Autodesk Fusion 360 part; units mm, degrees
(part 2 of 2)
sketch "Sketch40" plane through (15, 0, 0) normal (1, 0, 0) x (0, 1, 0)
  circle A0 centre (-253.0431, 52.1583) radius 1
  circle A1 centre (-244.4699, 38.6491) radius 1
  arc A2 (-251.4356, 49.6254) -> (-254.6506, 54.6913) centre (-253.0431, 52.1583) ccw
  line L0 (-254.6506, 54.6913) -> (-258.8722, 52.0122)
  line L1 (-258.8722, 52.0122) -> (-247.084, 33.437)
  line L2 (-247.084, 33.437) -> (-242.8624, 36.1161)
  arc A3 (-242.8624, 36.1161) -> (-246.0774, 41.1821) centre (-244.4699, 38.6491) ccw
  line L3 (-246.0774, 41.1821) -> (-251.4356, 49.6254)
  line L4 (-247.084, 33.437) -> (-258.8631, 51.9978)
  arc A4 (-258.8631, 51.9978) -> (-261.5307, 48.6113) centre (-254.1449, 45.5373) ccw
  line L5 (-261.5307, 48.6113) -> (-266.7096, 36.1683)
  arc A5 (-266.7096, 36.1683) -> (-267.0495, 31.0174) centre (-259.3238, 33.0942) ccw
  line L6 (-267.0495, 31.0174) -> (-253.1035, -20.86)
  arc A6 (-252.8389, -23.3324) -> (-253.1035, -20.86) centre (-260.8292, -22.9369) ccw
  line L7 (-252.8389, -23.3324) -> (-253.2356, -31.3463)
  arc A7 (-253.2356, -31.3463) -> (-251.6744, -33.3971) centre (-251.2381, -31.4452) ccw
  line L8 (-251.6744, -33.3971) -> (-249.3599, -33.9144)
  arc A8 (-249.3599, -33.9144) -> (-246.9237, -31.9835) centre (-248.9236, -31.9626) ccw
  line L9 (-246.9237, -31.9835) -> (-246.3282, 24.8623)
  arc A9 (-245.7143, 27.8528) -> (-246.3282, 24.8623) centre (-238.3286, 24.7785) ccw
  line L10 (-245.7143, 27.8528) -> (-241.7002, 37.4962)
  arc A10 (-242.8624, 36.1161) -> (-241.7002, 37.4962) centre (-244.4699, 38.6491) ccw
  line L11 (-242.8624, 36.1161) -> (-247.084, 33.437)
  circle A11 centre (-249.9129, -30.9524) radius 1
  circle A12 centre (-249.8605, -25.9531) radius 1
extrude "Extrude36" add sketch "Sketch40" along normal blind 3.5 bodies 4
sketch "Sketch41" plane through (15, 0, 0) normal (-1, 0, 0) x (0, -1, 0)
  arc A0 (241.7002, 37.4962) -> (242.8624, 36.1161) centre (244.4699, 38.6491) ccw
  line L0 (241.7002, 37.4962) -> (245.7143, 27.8528)
  arc A1 (246.3282, 24.8623) -> (245.7143, 27.8528) centre (238.3286, 24.7785) ccw
  line L1 (246.3282, 24.8623) -> (246.9237, -31.9835)
  arc A2 (246.9237, -31.9835) -> (249.3599, -33.9144) centre (248.9236, -31.9626) ccw
  line L2 (249.3599, -33.9144) -> (251.6744, -33.3971)
  arc A3 (251.6744, -33.3971) -> (253.2356, -31.3463) centre (251.2381, -31.4452) ccw
  line L3 (253.2356, -31.3463) -> (252.8389, -23.3324)
  arc A4 (253.1035, -20.86) -> (252.8389, -23.3324) centre (260.8292, -22.9369) ccw
  line L4 (253.1035, -20.86) -> (267.0495, 31.0174)
  arc A5 (267.0495, 31.0174) -> (266.7096, 36.1683) centre (259.3238, 33.0942) ccw
  line L5 (266.7096, 36.1683) -> (261.5307, 48.6113)
  arc A6 (261.5307, 48.6113) -> (258.8631, 51.9978) centre (254.1449, 45.5373) ccw
  line L6 (258.8631, 51.9978) -> (247.084, 33.437)
  line L7 (247.084, 33.437) -> (242.8624, 36.1161)
  circle A7 centre (249.9129, -30.9524) radius 1
  circle A8 centre (249.8605, -25.9531) radius 1
  line L8 (310.6552, -59.0578) -> (310.5183, -60.4688)
  line L9 (310.5183, -60.4688) -> (319.2523, -66.803)
  line L10 (319.2523, -66.803) -> (317.0688, -56.4133)
  line L11 (316.2366, -56.1583) -> (317.0688, -56.4133)
  circle A9 centre (229.817, 57.4821) radius 2.5
  circle A10 centre (206.2381, 18.5393) radius 2.5
  line L12 (305.328, 107.1994) -> (305.7767, 107.9451)
  line L13 (316.386, 107.5503) -> (305.7767, 107.9451)
  line L14 (306.791, 101.0823) -> (308.127, 100.6081)
  line L15 (308.127, 100.6081) -> (316.386, 107.5503)
  line L16 (253.1574, -29.8616) -> (253.7234, -30.5228)
  line L17 (250, -40.4651) -> (253.7234, -30.5228)
  line L18 (246.0196, -30.437) -> (250, -40.4651)
  line L19 (246.8913, -29.319) -> (246.0196, -30.437)
  line L20 (253.2296, -31.3409) -> (252.8387, -23.3266)
  line L21 (246.3626, 24.8727) -> (246.9172, -31.9735)
  line L22 (252.8387, -23.3266) -> (246.8357, -23.6195)
  line L23 (246.8357, -23.6195) -> (246.8913, -29.319)
  line L24 (252.8387, -23.3266) -> (253.1574, -29.8616)
  dimension "d299" = 76
  dimension "d301" = -108.4
  dimension "d308" = 250
  constraint coincident L21 L22.end
  constraint perpendicular L20 L22
  constraint parallel L21 L23
  constraint tangent A4 L24
  measures "d308" horizontal distance of L17.start origin
extrude "Extrude37" add sketch "Sketch41" along normal blind 30 contours L1 A2 L2 A3 L3 A4 L16 L20 L22 L24 | L1 A2 L2 A3 L3 L16 L17 L18 L19 L21 L23 bodies 4
sketch "Sketch42" plane through (0, 0, 0) normal (1, 0, 0) x (0, 1, 0)
  line L0 (-250.4928, -40.3888) -> (-250, -40.4732)
  line L1 (-250, -40.4732) -> (-249.5072, -40.5575)
  arc A0 (-250.4928, -40.3888) -> (-249.5072, -40.5575) centre (-250, -40.4732) ccw
  point P0 (-250, -40.4732)
  dimension "d305" = 1
  dimension "d307" = 250
  constraint coincident P0 L0.end
  constraint parallel L0 L1
  measures "d305" diameter of A0
  measures "d307" horizontal distance of origin L0.end
revolve "Revolve1" cut sketch "Sketch42" angle 360 about axis through (0, -250.4928, -40.3888) along (0, 0.985671, -0.168678) bodies 4
move_body "Move1" bodies 1 3 4 2 to x (1, 0, 0) y (0, 1, 0) z (0, 0, 1) at (0, 0, 59)
move_body "Move2" bodies 2 1 3 4 to x (1, 0, 0) y (0, 1, 0) z (0, 0, 1) at (0, 0, -18.535)
copy_body "Body->Comp5" bodies 2 removing the originals makes body 5 in component "coxa"
copy_body "Body->Comp6" bodies 1 removing the originals makes body 6 in component "base_link"
copy_body "Body->Comp7" bodies 3 removing the originals makes body 7 in component "femur"
copy_body "Body->Comp8" bodies 4 removing the originals makes body 8 in component "tibia"
component_pattern "component pattern"
component "base_link" placed x (1, 0, 0) y (0, 1, 0) z (0, 0, 1) at (0, 0, 0)
component "femur" placed x (1, 0, 0) y (0, 1, 0) z (0, 0, 1) at (0, 0, 0)
component "tibia" placed x (1, 0, 0) y (0, 1, 0) z (0, 0, 1) at (0, 0, 0)
component "coxa" placed x (1, 0, 0) y (0, 1, 0) z (0, 0, 1) at (0, 0, 0)
component "coxa" placed x (0.5, 0.866025, 0) y (-0.866025, 0.5, 0) z (0, 0, 1) at (0, 0, 0)
component "femur" placed x (0.5, 0.866025, 0) y (-0.866025, 0.5, 0) z (0, 0, 1) at (0, 0, 0)
component "tibia" placed x (0.5, 0.866025, 0) y (-0.866025, 0.5, 0) z (0, 0, 1) at (0, 0, 0)
component "coxa" placed x (-0.5, 0.866025, 0) y (-0.866025, -0.5, 0) z (0, 0, 1) at (0, 0, 0)
component "femur" placed x (-0.5, 0.866025, 0) y (-0.866025, -0.5, 0) z (0, 0, 1) at (0, 0, 0)
component "tibia" placed x (-0.5, 0.866025, 0) y (-0.866025, -0.5, 0) z (0, 0, 1) at (0, 0, 0)
component "coxa" placed x (-1, 0, 0) y (0, -1, 0) z (0, 0, 1) at (0, 0, 0)
component "femur" placed x (-1, 0, 0) y (0, -1, 0) z (0, 0, 1) at (0, 0, 0)
component "tibia" placed x (-1, 0, 0) y (0, -1, 0) z (0, 0, 1) at (0, 0, 0)
component "coxa" placed x (-0.5, -0.866025, 0) y (0.866025, -0.5, 0) z (0, 0, 1) at (0, 0, 0)
component "femur" placed x (-0.5, -0.866025, 0) y (0.866025, -0.5, 0) z (0, 0, 1) at (0, 0, 0)
component "tibia" placed x (-0.5, -0.866025, 0) y (0.866025, -0.5, 0) z (0, 0, 1) at (0, 0, 0)
component "coxa" placed x (0.5, -0.866025, 0) y (0.866025, 0.5, 0) z (0, 0, 1) at (0, 0, 0)
component "femur" placed x (0.5, -0.866025, 0) y (0.866025, 0.5, 0) z (0, 0, 1) at (0, 0, 0)
component "tibia" placed x (0.5, -0.866025, 0) y (0.866025, 0.5, 0) z (0, 0, 1) at (0, 0, 0)
equation "d51 = ( 5.8 * 2 ) * 1 mm"
equation "d81 = ( 37 / 2 ) * 1 mm"
equation "d103 = ( 5.8 * 2 ) * 1 mm"
equation "d239 = ( 7.8 * 2 ) * 1 mm"
equation "d250 = ( 28.712 * 2 ) * 1 mm"
equation "d258 = ( 7.8 * 2 ) * 1 mm"
